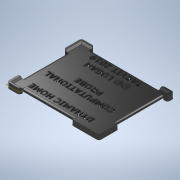
# Autodesk Inventor part: UNO Cover
Saved by Autodesk Inventor 2020.1 (Build 241239000, 239)
## iProperties
Created: 2019-09-15
Part Number: UNO Cover
Material: Generic
Document SubType Name: Modeling
Designer: Logan
Density: 1 g/cm^3
Appearance: Glossy - Black
Author: Logan
Autodesk Inventor part; units mm, degrees
(part 1 of 2)
ref_plane "YZ Plane" through (0, 0, 0) normal (1, 0, 0) x (0, 1, 0)
ref_plane "XZ Plane" through (0, 0, 0) normal (0, 1, 0) x (-1, 0, 0)
ref_plane "XY Plane" through (0, 0, 0) normal (0, 0, 1) x (1, 0, 0)
sketch "Sketch1" plane through (0, 0, 0) normal (0, 1, 0) x (-1, 0, 0)
  line L0 (0, 0) -> (-79.8, 0)
  line L1 (-79.8, 0) -> (-79.8, 63.434)
  line L2 (-79.8, 63.434) -> (0, 63.434)
  line L3 (0, 63.434) -> (0, 0)
  line L4 (-79.8, 0) -> (-73.207, 0)
  line L5 (-73.207, 0) -> (-73.207, 3)
  line L6 (-73.207, 3) -> (-79.8, 3)
  line L7 (-79.8, 3) -> (-79.8, 0)
  line L8 (-79.8, 63.434) -> (-76.8, 63.434)
  line L9 (-76.8, 63.434) -> (-76.8, 47.837)
  line L10 (-76.8, 47.837) -> (-79.8, 47.837)
  line L11 (-79.8, 47.837) -> (-79.8, 63.434)
  line L12 (-79.8, 63.434) -> (-57, 63.434)
  line L13 (-57, 63.434) -> (-57, 60.434)
  line L14 (-57, 60.434) -> (-79.8, 60.434)
  line L15 (-79.8, 60.434) -> (-79.8, 63.434)
  line L16 (-57, 63.434) -> (-31, 63.434)
  line L17 (-31, 63.434) -> (-31, 60.434)
  line L18 (-31, 60.434) -> (-57, 60.434)
  line L19 (-57, 60.434) -> (-57, 63.434)
  line L20 (-31, 60.434) -> (-29.5, 60.434)
  line L21 (-29.5, 60.434) -> (-29.5, 63.434)
  line L22 (-29.5, 63.434) -> (-31, 63.434)
  line L23 (-31, 63.434) -> (-31, 60.434)
  line L24 (0, 63.434) -> (-8.5, 63.434)
  line L25 (-8.5, 63.434) -> (-8.5, 60.434)
  line L26 (-8.5, 60.434) -> (0, 60.434)
  line L27 (0, 60.434) -> (0, 63.434)
  line L28 (0, 63.434) -> (-3, 63.434)
  line L29 (-3, 63.434) -> (-3, 55.505)
  line L30 (-3, 55.505) -> (0, 55.505)
  line L31 (0, 55.505) -> (0, 63.434)
  line L32 (0, 55.505) -> (-3, 55.505)
  line L33 (-3, 55.505) -> (-3, 46.153)
  line L34 (-3, 46.153) -> (0, 46.153)
  line L35 (0, 46.153) -> (0, 55.505)
  line L36 (-3, 46.153) -> (0, 46.153)
  line L37 (0, 46.153) -> (0, 40.598)
  line L38 (0, 40.598) -> (-3, 40.598)
  line L39 (-3, 40.598) -> (-3, 46.153)
  line L40 (0, 0) -> (-4.25, 0)
  line L41 (-4.25, 0) -> (-4.25, 13.458)
  line L42 (-4.25, 13.458) -> (0, 13.458)
  line L43 (0, 13.458) -> (0, 0)
  line L44 (0, 0) -> (-8.939, 0)
  line L45 (-8.939, 0) -> (-8.939, 3)
  line L46 (-8.939, 3) -> (0, 3)
  line L47 (0, 3) -> (0, 0)
  line L48 (-8.939, 0) -> (0, 0)
  line L49 (0, 0) -> (0, -3)
  line L50 (0, -3) -> (-8.939, -3)
  line L51 (-8.939, -3) -> (-8.939, 0)
  line L52 (0, -3) -> (3, -3)
  line L53 (3, -3) -> (3, 13.458)
  line L54 (3, 13.458) -> (0, 13.458)
  line L55 (0, 13.458) -> (0, -3)
  line L56 (0, 40.598) -> (3, 40.598)
  line L57 (3, 40.598) -> (3, 46.153)
  line L58 (3, 46.153) -> (0, 46.153)
  line L59 (0, 46.153) -> (0, 40.598)
  line L60 (0, 55.505) -> (3, 55.505)
  line L61 (3, 55.505) -> (3, 63.434)
  line L62 (3, 63.434) -> (0, 63.434)
  line L63 (0, 63.434) -> (0, 55.505)
  line L64 (-8.5, 63.434) -> (3, 63.434)
  line L65 (3, 63.434) -> (3, 66.434)
  line L66 (3, 66.434) -> (-8.5, 66.434)
  line L67 (-8.5, 66.434) -> (-8.5, 63.434)
  line L68 (-29.5, 63.434) -> (-31, 63.434)
  line L69 (-31, 63.434) -> (-31, 66.434)
  line L70 (-31, 66.434) -> (-29.5, 66.434)
  line L71 (-29.5, 66.434) -> (-29.5, 63.434)
  line L72 (-57, 63.434) -> (-79.8, 63.434)
  line L73 (-79.8, 63.434) -> (-79.8, 66.434)
  line L74 (-79.8, 66.434) -> (-57, 66.434)
  line L75 (-57, 66.434) -> (-57, 63.434)
  line L76 (-79.8, 66.434) -> (-82.8, 66.434)
  line L77 (-82.8, 66.434) -> (-82.8, 47.837)
  line L78 (-82.8, 47.837) -> (-79.8, 47.837)
  line L79 (-79.8, 47.837) -> (-79.8, 66.434)
  line L80 (-79.8, 3) -> (-83.6566, 3)
  line L81 (-83.6566, 3) -> (-83.6566, 0)
  line L82 (-83.6566, 0) -> (-79.8, 0)
  line L83 (-79.8, 0) -> (-79.8, 3)
  line L84 (-83.6566, 0) -> (-73.207, 0)
  line L85 (-73.207, 0) -> (-73.207, -3)
  line L86 (-73.207, -3) -> (-83.6566, -3)
  line L87 (-83.6566, -3) -> (-83.6566, 0)
  dimension "d0" = 79.8
  dimension "d1" = 63.434
  dimension "d2" = 6.593
  dimension "d3" = 3
  dimension "d4" = 3
  dimension "d5" = 15.597
  dimension "d6" = 22.8
  dimension "d7" = 3
  dimension "d8" = 26
  dimension "d9" = 1.5
  dimension "d10" = 8.5
  dimension "d11" = 3
  dimension "d12" = 7.929
  dimension "d13" = 9.352
  dimension "d14" = 5.555
  dimension "d15" = 13.458
  dimension "d16" = 8.939
  dimension "d17" = 3
  dimension "d18" = 3
  dimension "d19" = 3
  dimension "d20" = 3
  dimension "d21" = 3
  dimension "d22" = 11.5
  dimension "d23" = 3
  dimension "d24" = 3
  constraints: 176 end point, 44 parallel, 22 horizontal, 22 perpendicular, 6 point on line
  measures "d0" distance of L1.end L2.end
  measures "d1" distance of L0.end L1.end
  measures "d2" distance of L6.end L5.end
  measures "d3" distance of L5.end L4.end
  measures "d4" distance of L9.end L10.end
  measures "d5" distance of L8.end L9.end
  measures "d6" distance of L13.end L14.end
  measures "d7" distance of L12.end L13.end
  measures "d8" distance of L17.end L18.end
  measures "d9" distance of L22.end L21.end
  measures "d10" distance of L26.end L25.end
  measures "d11" distance of L30.end L29.end
  measures "d12" distance of L29.end L28.end
  measures "d13" distance of L33.end L32.end
  measures "d14" distance of L36.end L37.end
  measures "d15" distance of L40.end L41.end
  measures "d16" distance of L45.end L46.end
  measures "d17" distance of L44.end L45.end
  measures "d18" distance of L48.end L49.end
  measures "d19" distance of L54.end L53.end
  measures "d20" distance of L58.end L57.end
  measures "d21" distance of L62.end L61.end
  measures "d22" distance of L66.end L65.end
  measures "d23" distance of L65.end L64.end
  measures "d24" distance of L78.end L77.end
extrude "Extrusion1" add sketch "Sketch1" against normal mid plane 5 contours L49 L50 L51 L0 | L3 L54 L53 L52 L49 | L85 L86 L87 L82 L0 | L82 L81 L80 L1 | L3 L62 L61 L60 | L78 L77 L76 L73 L1 | L2 L67 L66 L65 L62 | L73 L74 L75 L2
ref_plane "Work Plane1" through (0, 0, 0) normal (0, 1, 0) x (1, 0, 0)
sketch "Sketch2" plane through (0, 0, 0) normal (0, 1, 0) x (1, 0, 0)
  line L0 (0, -63.434) -> (8.5, -63.434) projected
  line L1 (79.8, 0) -> (73.207, 0) projected
  line L2 (0, -63.434) -> (79.8, -63.434)
  line L3 (79.8, -63.434) -> (79.8, 0)
  line L4 (79.8, 0) -> (0, 0)
  line L5 (0, 0) -> (0, -63.434)
  constraints: 8 end point, 2 parallel, 1 horizontal, 1 perpendicular
extrude "Extrusion2" add sketch "Sketch2" against normal mid plane 2
fillet "Fillet1" radius 2 16 edges at (82.8, 0, 66.434) (-3, 0, 66.434) (-3, 0, -3) (83.6566, 0, -3) (82.8, 0, 47.837) (8.5, 0, 66.434) (-3, 0, 55.505) (8.939, 0, -3) (73.207, 0, -3) (83.6566, 0, 3) (57, 0, 66.434) (-3, 0, 13.458) (79.8, 1, 25.4185) (41.073, 1, 0) (0, 1, 34.4815) (32.75, 1, 63.434)
chamfer "Chamfer1" distance 1.5 angle 45 2 edges at (79.8, 2.5, 55.6355) (68.4, 2.5, 63.434)
chamfer "Chamfer2" distance 1.5 angle 45 6 edges at (79.8, 2.5, 1.5) (76.5035, 2.5, 0) (4.4695, 2.5, 0) (0, 2.5, 6.729) (0, 2.5, 59.4695) (4.25, 2.5, 63.434)
sketch "Sketch3" plane through (0, 1, 0) normal (0, 1, 0) x (1, 0, 0)
  line L0 (67.7847, -38.7304) -> (8.3805, -38.7304) construction
  line L1 (8.3805, -38.7304) -> (8.3805, -23.3742) construction
  line L2 (8.3805, -23.3742) -> (67.7847, -23.3742) construction
  line L3 (67.7847, -23.3742) -> (67.7847, -38.7304) construction
  spline S0 degree 2 poles (62.4497, -56.7331) (62.4497, -56.0041) (63.086, -54.8579) (63.5706, -54.5503) knots 0 0 0 1 2 2 2
  spline S1 degree 2 poles (63.5706, -54.5503) (63.9752, -54.289) (64.9275, -54.1373) (65.4627, -54.1373) knots 0 0 0 1 2 2 2
  line L4 (65.4627, -54.1373) -> (67.0893, -54.1373)
  line L5 (67.0893, -54.1373) -> (67.0893, -59.3373)
  line L6 (67.0893, -59.3373) -> (65.4795, -59.3373)
  spline S2 degree 2 poles (65.4795, -59.3373) (64.9317, -59.3373) (63.9752, -59.1982) (63.5538, -58.9285) knots 0 0 0 1 2 2 2
  spline S3 degree 2 poles (63.5538, -58.9285) (63.0439, -58.5998) (62.4497, -57.4874) (62.4497, -56.7331) knots 0 0 0 1 2 2 2
  spline S4 degree 2 poles (63.7897, -56.7415) (63.7897, -57.2556) (64.1437, -57.9888) (64.5061, -58.1953) knots 0 0 0 1 2 2 2
  spline S5 degree 2 poles (64.5061, -58.1953) (64.7716, -58.3386) (65.3531, -58.3681) (65.7577, -58.3681) knots 0 0 0 1 2 2 2
  line L7 (65.7577, -58.3681) -> (65.7829, -58.3681)
  line L8 (65.7829, -58.3681) -> (65.7829, -55.1107)
  line L9 (65.7829, -55.1107) -> (65.7577, -55.1107)
  spline S6 degree 2 poles (65.7577, -55.1107) (65.3194, -55.1107) (64.7168, -55.1402) (64.4429, -55.313) knots 0 0 0 1 2 2 2
  spline S7 degree 2 poles (64.4429, -55.313) (64.1226, -55.5152) (63.7897, -56.2274) (63.7897, -56.7415) knots 0 0 0 1 2 2 2
  line L10 (57.3508, -59.3373) -> (59.146, -56.3075)
  line L11 (59.146, -56.3075) -> (59.146, -54.1373)
  line L12 (59.146, -54.1373) -> (60.4523, -54.1373)
  line L13 (60.4523, -54.1373) -> (60.4523, -56.2443)
  line L14 (60.4523, -56.2443) -> (62.2769, -59.3373)
  line L15 (62.2769, -59.3373) -> (60.7894, -59.3373)
  line L16 (60.7894, -59.3373) -> (59.7739, -57.4832)
  line L17 (59.7739, -57.4832) -> (58.792, -59.3373)
  line L18 (58.792, -59.3373) -> (57.3508, -59.3373)
  line L19 (52.4248, -54.1373) -> (53.6805, -54.1373)
  line L20 (53.6805, -54.1373) -> (55.6863, -57.7613)
  line L21 (55.6863, -57.7613) -> (55.6863, -54.1373)
  line L22 (55.6863, -54.1373) -> (56.8789, -54.1373)
  line L23 (56.8789, -54.1373) -> (56.8789, -59.3373)
  line L24 (56.8789, -59.3373) -> (55.2776, -59.3373)
  line L25 (55.2776, -59.3373) -> (53.6173, -56.358)
  line L26 (53.6173, -56.358) -> (53.6173, -59.3373)
  line L27 (53.6173, -59.3373) -> (52.4248, -59.3373)
  line L28 (52.4248, -59.3373) -> (52.4248, -54.1373)
  line L29 (51.9275, -54.1373) -> (50.1703, -59.3373)
  line L30 (50.1703, -59.3373) -> (48.746, -59.3373)
  line L31 (48.746, -59.3373) -> (46.9888, -54.1373)
  line L32 (46.9888, -54.1373) -> (48.333, -54.1373)
  line L33 (48.333, -54.1373) -> (48.6575, -55.1992)
  line L34 (48.6575, -55.1992) -> (50.2925, -55.1992)
  line L35 (50.2925, -55.1992) -> (50.6212, -54.1373)
  line L36 (50.6212, -54.1373) -> (51.9275, -54.1373)
  line L37 (48.944, -56.1431) -> (49.475, -57.8624)
  line L38 (49.475, -57.8624) -> (50.0102, -56.1431)
  line L39 (50.0102, -56.1431) -> (48.944, -56.1431)
  line L40 (41.1609, -54.1373) -> (42.4588, -54.1373)
  line L41 (42.4588, -54.1373) -> (42.4588, -57.5843)
  line L42 (42.4588, -57.5843) -> (43.4027, -55.3593)
  line L43 (43.4027, -55.3593) -> (44.2961, -55.3593)
  line L44 (44.2961, -55.3593) -> (45.24, -57.5843)
  line L45 (45.24, -57.5843) -> (45.24, -54.1373)
  line L46 (45.24, -54.1373) -> (46.4705, -54.1373)
  line L47 (46.4705, -54.1373) -> (46.4705, -59.3373)
  line L48 (46.4705, -59.3373) -> (44.9661, -59.3373)
  line L49 (44.9661, -59.3373) -> (43.8115, -56.771)
  line L50 (43.8115, -56.771) -> (42.6653, -59.3373)
  line L51 (42.6653, -59.3373) -> (41.1609, -59.3373)
  line L52 (41.1609, -59.3373) -> (41.1609, -54.1373)
  line L53 (37.4948, -54.1373) -> (40.2928, -54.1373)
  line L54 (40.2928, -54.1373) -> (40.2928, -55.0433)
  line L55 (40.2928, -55.0433) -> (39.547, -55.0433)
  line L56 (39.547, -55.0433) -> (39.547, -58.4313)
  line L57 (39.547, -58.4313) -> (40.2928, -58.4313)
  line L58 (40.2928, -58.4313) -> (40.2928, -59.3373)
  line L59 (40.2928, -59.3373) -> (37.4948, -59.3373)
  line L60 (37.4948, -59.3373) -> (37.4948, -58.4313)
  line L61 (37.4948, -58.4313) -> (38.2406, -58.4313)
  line L62 (38.2406, -58.4313) -> (38.2406, -55.0433)
  line L63 (38.2406, -55.0433) -> (37.4948, -55.0433)
  line L64 (37.4948, -55.0433) -> (37.4948, -54.1373)
  spline S8 degree 2 poles (34.3849, -54.0362) (35.5564, -54.0362) (36.9301, -55.452) (36.9301, -56.7331) knots 0 0 0 1 2 2 2
  spline S9 degree 2 poles (36.9301, -56.7331) (36.9301, -57.9678) (35.5521, -59.4384) (34.3807, -59.4384) knots 0 0 0 1 2 2 2
  spline S10 degree 2 poles (34.3807, -59.4384) (34.073, -59.4384) (33.5758, -59.3668) (33.3483, -59.3078) knots 0 0 0 1 2 2 2
  spline S11 degree 2 poles (33.3483, -59.3078) (33.1713, -59.253) (32.7541, -59.0718) (32.6235, -59.0044) knots 0 0 0 1 2 2 2
  line L65 (32.6235, -59.0044) -> (32.6235, -57.7655)
  line L66 (32.6235, -57.7655) -> (32.7541, -57.7655)
  spline S12 degree 2 poles (32.7541, -57.7655) (32.851, -57.8498) (33.1376, -58.0857) (33.3188, -58.1953) knots 0 0 0 1 2 2 2
  spline S13 degree 2 poles (33.3188, -58.1953) (33.5, -58.3091) (33.934, -58.465) (34.1742, -58.465) knots 0 0 0 1 2 2 2
  spline S14 degree 2 poles (34.1742, -58.465) (34.4565, -58.465) (34.9243, -58.288) (35.1392, -58.0647) knots 0 0 0 1 2 2 2
  spline S15 degree 2 poles (35.1392, -58.0647) (35.333, -57.8666) (35.5816, -57.1882) (35.5816, -56.7289) knots 0 0 0 1 2 2 2
  spline S16 degree 2 poles (35.5816, -56.7289) (35.5816, -56.2443) (35.3246, -55.5827) (35.1139, -55.3804) knots 0 0 0 1 2 2 2
  spline S17 degree 2 poles (35.1139, -55.3804) (34.9116, -55.1823) (34.4144, -55.0096) (34.1658, -55.0096) knots 0 0 0 1 2 2 2
  spline S18 degree 2 poles (34.1658, -55.0096) (33.9087, -55.0096) (33.441, -55.1823) (33.2808, -55.2877) knots 0 0 0 1 2 2 2
  spline S19 degree 2 poles (33.2808, -55.2877) (33.1038, -55.393) (32.8384, -55.6164) (32.7414, -55.7049) knots 0 0 0 1 2 2 2
  line L67 (32.7414, -55.7049) -> (32.6235, -55.7049)
  line L68 (32.6235, -55.7049) -> (32.6235, -54.4828)
  spline S20 degree 2 poles (32.6235, -54.4828) (32.7667, -54.4154) (33.1418, -54.2469) (33.344, -54.1879) knots 0 0 0 1 2 2 2
  spline S21 degree 2 poles (33.344, -54.1879) (33.5884, -54.112) (34.0141, -54.0362) (34.3849, -54.0362) knots 0 0 0 1 2 2 2
  line L69 (25.3713, -54.1373) -> (26.6776, -54.1373)
  line L70 (26.6776, -54.1373) -> (26.6776, -56.4423)
  line L71 (26.6776, -56.4423) -> (28.4517, -56.4423)
  line L72 (28.4517, -56.4423) -> (28.4517, -54.1373)
  line L73 (28.4517, -54.1373) -> (29.758, -54.1373)
  line L74 (29.758, -54.1373) -> (29.758, -59.3373)
  line L75 (29.758, -59.3373) -> (28.4517, -59.3373)
  line L76 (28.4517, -59.3373) -> (28.4517, -57.4326)
  line L77 (28.4517, -57.4326) -> (26.6776, -57.4326)
  line L78 (26.6776, -57.4326) -> (26.6776, -59.3373)
  line L79 (26.6776, -59.3373) -> (25.3713, -59.3373)
  line L80 (25.3713, -59.3373) -> (25.3713, -54.1373)
  spline S22 degree 2 poles (19.5602, -56.7373) (19.5602, -55.4731) (20.9087, -54.0277) (22.0802, -54.0277) knots 0 0 0 1 2 2 2
  spline S23 degree 2 poles (22.0802, -54.0277) (23.2559, -54.0277) (24.5959, -55.49) (24.5959, -56.7373) knots 0 0 0 1 2 2 2
  spline S24 degree 2 poles (24.5959, -56.7373) (24.5959, -57.9888) (23.2559, -59.4469) (22.0802, -59.4469) knots 0 0 0 1 2 2 2
  spline S25 degree 2 poles (22.0802, -59.4469) (20.9087, -59.4469) (19.5602, -57.9973) (19.5602, -56.7373) knots 0 0 0 1 2 2 2
  spline S26 degree 2 poles (20.9087, -56.7373) (20.9087, -57.205) (21.0983, -57.8582) (21.2627, -58.0647) knots 0 0 0 1 2 2 2
  spline S27 degree 2 poles (21.2627, -58.0647) (21.427, -58.2796) (21.8484, -58.465) (22.076, -58.465) knots 0 0 0 1 2 2 2
  spline S28 degree 2 poles (22.076, -58.465) (22.3162, -58.465) (22.7081, -58.2922) (22.8893, -58.0731) knots 0 0 0 1 2 2 2
  spline S29 degree 2 poles (22.8893, -58.0731) (23.0494, -57.8708) (23.2474, -57.2008) (23.2474, -56.7373) knots 0 0 0 1 2 2 2
  spline S30 degree 2 poles (23.2474, -56.7373) (23.2474, -56.2569) (23.0578, -55.6248) (22.8935, -55.4099) knots 0 0 0 1 2 2 2
  spline S31 degree 2 poles (22.8935, -55.4099) (22.7291, -55.195) (22.3035, -55.0096) (22.076, -55.0096) knots 0 0 0 1 2 2 2
  spline S32 degree 2 poles (22.076, -55.0096) (21.8442, -55.0096) (21.4144, -55.2076) (21.2585, -55.4183) knots 0 0 0 1 2 2 2
  spline S33 degree 2 poles (21.2585, -55.4183) (21.0899, -55.6459) (20.9087, -56.2485) (20.9087, -56.7373) knots 0 0 0 1 2 2 2
  line L81 (13.4753, -54.1373) -> (14.7732, -54.1373)
  line L82 (14.7732, -54.1373) -> (14.7732, -57.5843)
  line L83 (14.7732, -57.5843) -> (15.7171, -55.3593)
  line L84 (15.7171, -55.3593) -> (16.6105, -55.3593)
  line L85 (16.6105, -55.3593) -> (17.5544, -57.5843)
  line L86 (17.5544, -57.5843) -> (17.5544, -54.1373)
  line L87 (17.5544, -54.1373) -> (18.7849, -54.1373)
  line L88 (18.7849, -54.1373) -> (18.7849, -59.3373)
  line L89 (18.7849, -59.3373) -> (17.2805, -59.3373)
  line L90 (17.2805, -59.3373) -> (16.1259, -56.771)
  line L91 (16.1259, -56.771) -> (14.9797, -59.3373)
  line L92 (14.9797, -59.3373) -> (13.4753, -59.3373)
  line L93 (13.4753, -59.3373) -> (13.4753, -54.1373)
  line L94 (12.3966, -54.1373) -> (12.3966, -59.3373)
  line L95 (12.3966, -59.3373) -> (8.8821, -59.3373)
  line L96 (8.8821, -59.3373) -> (8.8821, -58.347)
  line L97 (8.8821, -58.347) -> (11.0987, -58.347)
  line L98 (11.0987, -58.347) -> (11.0987, -57.4326)
  line L99 (11.0987, -57.4326) -> (9.0549, -57.4326)
  line L100 (9.0549, -57.4326) -> (9.0549, -56.4423)
  line L101 (9.0549, -56.4423) -> (11.0987, -56.4423)
  line L102 (11.0987, -56.4423) -> (11.0987, -55.1276)
  line L103 (11.0987, -55.1276) -> (8.8821, -55.1276)
  line L104 (8.8821, -55.1276) -> (8.8821, -54.1373)
  line L105 (8.8821, -54.1373) -> (12.3966, -54.1373)
  spline S34 degree 2 poles (67.1862, -36.9128) (68.3577, -36.9128) (69.7314, -38.3287) (69.7314, -39.6097) knots 0 0 0 1 2 2 2
  spline S35 degree 2 poles (69.7314, -39.6097) (69.7314, -40.8444) (68.3534, -42.3151) (67.182, -42.3151) knots 0 0 0 1 2 2 2
  spline S36 degree 2 poles (67.182, -42.3151) (66.8743, -42.3151) (66.3771, -42.2435) (66.1495, -42.1845) knots 0 0 0 1 2 2 2
  spline S37 degree 2 poles (66.1495, -42.1845) (65.9726, -42.1297) (65.5554, -41.9485) (65.4248, -41.8811) knots 0 0 0 1 2 2 2
  line L106 (65.4248, -41.8811) -> (65.4248, -40.6422)
  line L107 (65.4248, -40.6422) -> (65.5554, -40.6422)
  spline S38 degree 2 poles (65.5554, -40.6422) (65.6523, -40.7264) (65.9389, -40.9624) (66.1201, -41.072) knots 0 0 0 1 2 2 2
  spline S39 degree 2 poles (66.1201, -41.072) (66.3013, -41.1858) (66.7353, -41.3417) (66.9755, -41.3417) knots 0 0 0 1 2 2 2
  spline S40 degree 2 poles (66.9755, -41.3417) (67.2578, -41.3417) (67.7256, -41.1647) (67.9405, -40.9414) knots 0 0 0 1 2 2 2
  spline S41 degree 2 poles (67.9405, -40.9414) (68.1343, -40.7433) (68.3829, -40.0649) (68.3829, -39.6055) knots 0 0 0 1 2 2 2
  spline S42 degree 2 poles (68.3829, -39.6055) (68.3829, -39.1209) (68.1259, -38.4593) (67.9152, -38.2571) knots 0 0 0 1 2 2 2
  spline S43 degree 2 poles (67.9152, -38.2571) (67.7129, -38.059) (67.2157, -37.8862) (66.9671, -37.8862) knots 0 0 0 1 2 2 2
  spline S44 degree 2 poles (66.9671, -37.8862) (66.71, -37.8862) (66.2423, -38.059) (66.0821, -38.1644) knots 0 0 0 1 2 2 2
  spline S45 degree 2 poles (66.0821, -38.1644) (65.9051, -38.2697) (65.6397, -38.4931) (65.5427, -38.5815) knots 0 0 0 1 2 2 2
  line L108 (65.5427, -38.5815) -> (65.4248, -38.5815)
  line L109 (65.4248, -38.5815) -> (65.4248, -37.3595)
  spline S46 degree 2 poles (65.4248, -37.3595) (65.568, -37.2921) (65.9431, -37.1235) (66.1453, -37.0645) knots 0 0 0 1 2 2 2
  spline S47 degree 2 poles (66.1453, -37.0645) (66.3897, -36.9887) (66.8154, -36.9128) (67.1862, -36.9128) knots 0 0 0 1 2 2 2
  spline S48 degree 2 poles (59.9213, -39.614) (59.9213, -38.3498) (61.2698, -36.9044) (62.4413, -36.9044) knots 0 0 0 1 2 2 2
  spline S49 degree 2 poles (62.4413, -36.9044) (63.617, -36.9044) (64.957, -38.3666) (64.957, -39.614) knots 0 0 0 1 2 2 2
  spline S50 degree 2 poles (64.957, -39.614) (64.957, -40.8655) (63.617, -42.3235) (62.4413, -42.3235) knots 0 0 0 1 2 2 2
  spline S51 degree 2 poles (62.4413, -42.3235) (61.2698, -42.3235) (59.9213, -40.8739) (59.9213, -39.614) knots 0 0 0 1 2 2 2
  spline S52 degree 2 poles (61.2698, -39.614) (61.2698, -40.0817) (61.4594, -40.7349) (61.6238, -40.9414) knots 0 0 0 1 2 2 2
  spline S53 degree 2 poles (61.6238, -40.9414) (61.7881, -41.1563) (62.2095, -41.3417) (62.4371, -41.3417) knots 0 0 0 1 2 2 2
  spline S54 degree 2 poles (62.4371, -41.3417) (62.6773, -41.3417) (63.0692, -41.1689) (63.2504, -40.9498) knots 0 0 0 1 2 2 2
  spline S55 degree 2 poles (63.2504, -40.9498) (63.4105, -40.7475) (63.6085, -40.0775) (63.6085, -39.614) knots 0 0 0 1 2 2 2
  spline S56 degree 2 poles (63.6085, -39.614) (63.6085, -39.1336) (63.4189, -38.5015) (63.2546, -38.2866) knots 0 0 0 1 2 2 2
  spline S57 degree 2 poles (63.2546, -38.2866) (63.0902, -38.0717) (62.6646, -37.8862) (62.4371, -37.8862) knots 0 0 0 1 2 2 2
  spline S58 degree 2 poles (62.4371, -37.8862) (62.2053, -37.8862) (61.7755, -38.0843) (61.6196, -38.295) knots 0 0 0 1 2 2 2
  spline S59 degree 2 poles (61.6196, -38.295) (61.451, -38.5226) (61.2698, -39.1251) (61.2698, -39.614) knots 0 0 0 1 2 2 2
  line L110 (53.8364, -37.014) -> (55.1343, -37.014)
  line L111 (55.1343, -37.014) -> (55.1343, -40.461)
  line L112 (55.1343, -40.461) -> (56.0782, -38.236)
  line L113 (56.0782, -38.236) -> (56.9716, -38.236)
  line L114 (56.9716, -38.236) -> (57.9155, -40.461)
  line L115 (57.9155, -40.461) -> (57.9155, -37.014)
  line L116 (57.9155, -37.014) -> (59.146, -37.014)
  line L117 (59.146, -37.014) -> (59.146, -42.214)
  line L118 (59.146, -42.214) -> (57.6416, -42.214)
  line L119 (57.6416, -42.214) -> (56.487, -39.6477)
  line L120 (56.487, -39.6477) -> (55.3408, -42.214)
  line L121 (55.3408, -42.214) -> (53.8364, -42.214)
  line L122 (53.8364, -42.214) -> (53.8364, -37.014)
  spline S60 degree 2 poles (48.7586, -40.5747) (48.7586, -40.2123) (48.9904, -39.555) (49.2053, -39.3358) knots 0 0 0 1 2 2 2
  spline S61 degree 2 poles (49.2053, -39.3358) (49.3359, -39.1968) (49.6562, -38.9692) (49.8458, -38.8892) knots 0 0 0 1 2 2 2
  spline S62 degree 2 poles (49.8458, -38.8892) (50.0397, -38.8091) (50.4906, -38.7164) (50.7687, -38.7164) knots 0 0 0 1 2 2 2
  line L123 (50.7687, -38.7164) -> (51.4513, -38.7164)
  line L124 (51.4513, -38.7164) -> (51.4513, -37.014)
  line L125 (51.4513, -37.014) -> (52.7577, -37.014)
  line L126 (52.7577, -37.014) -> (52.7577, -42.214)
  line L127 (52.7577, -42.214) -> (50.7392, -42.214)
  spline S63 degree 2 poles (50.7392, -42.214) (50.2925, -42.214) (49.6393, -42.0496) (49.3739, -41.8726) knots 0 0 0 1 2 2 2
  spline S64 degree 2 poles (49.3739, -41.8726) (49.0789, -41.6746) (48.7586, -41.0256) (48.7586, -40.5747) knots 0 0 0 1 2 2 2
  spline S65 degree 2 poles (50.0987, -40.541) (50.0987, -40.7644) (50.3094, -41.0804) (50.4526, -41.1394) knots 0 0 0 1 2 2 2
  spline S66 degree 2 poles (50.4526, -41.1394) (50.638, -41.2195) (50.9752, -41.2448) (51.2659, -41.2448) knots 0 0 0 1 2 2 2
  line L128 (51.2659, -41.2448) -> (51.4513, -41.2448)
  line L129 (51.4513, -41.2448) -> (51.4513, -39.6856)
  line L130 (51.4513, -39.6856) -> (51.3586, -39.6856)
  spline S67 degree 2 poles (51.3586, -39.6856) (51.1774, -39.6856) (50.8487, -39.694) (50.7265, -39.7151) knots 0 0 0 1 2 2 2
  spline S68 degree 2 poles (50.7265, -39.7151) (50.6212, -39.732) (50.3894, -39.8331) (50.3262, -39.8963) knots 0 0 0 1 2 2 2
  spline S69 degree 2 poles (50.3262, -39.8963) (50.1914, -40.0227) (50.0987, -40.305) (50.0987, -40.541) knots 0 0 0 1 2 2 2
  spline S70 degree 2 poles (45.9564, -36.9044) (47.0056, -36.9044) (48.135, -37.9157) (48.135, -38.8934) knots 0 0 0 1 2 2 2
  line L131 (48.135, -38.8934) -> (48.135, -42.214)
  line L132 (48.135, -42.214) -> (46.8286, -42.214)
  line L133 (46.8286, -42.214) -> (46.8286, -38.9692)
  spline S71 degree 2 poles (46.8286, -38.9692) (46.8286, -38.4256) (46.4199, -37.8947) (45.9564, -37.8947) knots 0 0 0 1 2 2 2
  spline S72 degree 2 poles (45.9564, -37.8947) (45.5055, -37.8947) (45.0841, -38.4046) (45.0841, -38.9692) knots 0 0 0 1 2 2 2
  line L134 (45.0841, -38.9692) -> (45.0841, -42.214)
  line L135 (45.0841, -42.214) -> (43.7778, -42.214)
  line L136 (43.7778, -42.214) -> (43.7778, -38.8976)
  spline S73 degree 2 poles (43.7778, -38.8976) (43.7778, -37.9368) (44.8776, -36.9044) (45.9564, -36.9044) knots 0 0 0 1 2 2 2
  line L137 (41.7761, -37.014) -> (41.7761, -41.2237)
  line L138 (41.7761, -41.2237) -> (43.3142, -41.2237)
  line L139 (43.3142, -41.2237) -> (43.3142, -42.214)
  line L140 (43.3142, -42.214) -> (38.9317, -42.214)
  line L141 (38.9317, -42.214) -> (38.9317, -41.2237)
  line L142 (38.9317, -41.2237) -> (40.4698, -41.2237)
  line L143 (40.4698, -41.2237) -> (40.4698, -37.014)
  line L144 (40.4698, -37.014) -> (41.7761, -37.014)
  line L145 (38.957, -37.014) -> (37.1998, -42.214)
  line L146 (37.1998, -42.214) -> (35.7755, -42.214)
  line L147 (35.7755, -42.214) -> (34.0183, -37.014)
  line L148 (34.0183, -37.014) -> (35.3625, -37.014)
  line L149 (35.3625, -37.014) -> (35.687, -38.0759)
  line L150 (35.687, -38.0759) -> (37.322, -38.0759)
  line L151 (37.322, -38.0759) -> (37.6507, -37.014)
  line L152 (37.6507, -37.014) -> (38.957, -37.014)
  line L153 (35.9735, -39.0198) -> (36.5045, -40.7391)
  line L154 (36.5045, -40.7391) -> (37.0397, -39.0198)
  line L155 (37.0397, -39.0198) -> (35.9735, -39.0198)
  line L156 (32.5013, -37.014) -> (32.5013, -41.2237)
  line L157 (32.5013, -41.2237) -> (34.0393, -41.2237)
  line L158 (34.0393, -41.2237) -> (34.0393, -42.214)
  line L159 (34.0393, -42.214) -> (29.6568, -42.214)
  line L160 (29.6568, -42.214) -> (29.6568, -41.2237)
  line L161 (29.6568, -41.2237) -> (31.1949, -41.2237)
  line L162 (31.1949, -41.2237) -> (31.1949, -37.014)
  line L163 (31.1949, -37.014) -> (32.5013, -37.014)
  line L164 (26.5343, -37.014) -> (29.3324, -37.014)
  line L165 (29.3324, -37.014) -> (29.3324, -37.92)
  line L166 (29.3324, -37.92) -> (28.5865, -37.92)
  line L167 (28.5865, -37.92) -> (28.5865, -41.308)
  line L168 (28.5865, -41.308) -> (29.3324, -41.308)
  line L169 (29.3324, -41.308) -> (29.3324, -42.214)
  line L170 (29.3324, -42.214) -> (26.5343, -42.214)
  line L171 (26.5343, -42.214) -> (26.5343, -41.308)
  line L172 (26.5343, -41.308) -> (27.2802, -41.308)
  line L173 (27.2802, -41.308) -> (27.2802, -37.92)
  line L174 (27.2802, -37.92) -> (26.5343, -37.92)
  line L175 (26.5343, -37.92) -> (26.5343, -37.014)
  spline S74 degree 2 poles (20.934, -39.614) (20.934, -38.3498) (22.2825, -36.9044) (23.4539, -36.9044) knots 0 0 0 1 2 2 2
  spline S75 degree 2 poles (23.4539, -36.9044) (24.6296, -36.9044) (25.9696, -38.3666) (25.9696, -39.614) knots 0 0 0 1 2 2 2
  spline S76 degree 2 poles (25.9696, -39.614) (25.9696, -40.8655) (24.6296, -42.3235) (23.4539, -42.3235) knots 0 0 0 1 2 2 2
  spline S77 degree 2 poles (23.4539, -42.3235) (22.2825, -42.3235) (20.934, -40.8739) (20.934, -39.614) knots 0 0 0 1 2 2 2
  spline S78 degree 2 poles (22.2825, -39.614) (22.2825, -40.0817) (22.4721, -40.7349) (22.6364, -40.9414) knots 0 0 0 1 2 2 2
  spline S79 degree 2 poles (22.6364, -40.9414) (22.8008, -41.1563) (23.2222, -41.3417) (23.4497, -41.3417) knots 0 0 0 1 2 2 2
  spline S80 degree 2 poles (23.4497, -41.3417) (23.6899, -41.3417) (24.0818, -41.1689) (24.263, -40.9498) knots 0 0 0 1 2 2 2
  spline S81 degree 2 poles (24.263, -40.9498) (24.4231, -40.7475) (24.6212, -40.0775) (24.6212, -39.614) knots 0 0 0 1 2 2 2
  spline S82 degree 2 poles (24.6212, -39.614) (24.6212, -39.1336) (24.4316, -38.5015) (24.2672, -38.2866) knots 0 0 0 1 2 2 2
  spline S83 degree 2 poles (24.2672, -38.2866) (24.1029, -38.0717) (23.6773, -37.8862) (23.4497, -37.8862) knots 0 0 0 1 2 2 2
  spline S84 degree 2 poles (23.4497, -37.8862) (23.2179, -37.8862) (22.7881, -38.0843) (22.6322, -38.295) knots 0 0 0 1 2 2 2
  spline S85 degree 2 poles (22.6322, -38.295) (22.4637, -38.5226) (22.2825, -39.1251) (22.2825, -39.614) knots 0 0 0 1 2 2 2
  line L176 (15.7045, -37.014) -> (16.9602, -37.014)
  line L177 (16.9602, -37.014) -> (18.9661, -40.638)
  line L178 (18.9661, -40.638) -> (18.9661, -37.014)
  line L179 (18.9661, -37.014) -> (20.1586, -37.014)
  line L180 (20.1586, -37.014) -> (20.1586, -42.214)
  line L181 (20.1586, -42.214) -> (18.5573, -42.214)
  line L182 (18.5573, -42.214) -> (16.897, -39.2347)
  line L183 (16.897, -39.2347) -> (16.897, -42.214)
  line L184 (16.897, -42.214) -> (15.7045, -42.214)
  line L185 (15.7045, -42.214) -> (15.7045, -37.014)
  line L186 (15.2072, -37.014) -> (13.45, -42.214)
  line L187 (13.45, -42.214) -> (12.0257, -42.214)
  line L188 (12.0257, -42.214) -> (10.2685, -37.014)
  line L189 (10.2685, -37.014) -> (11.6128, -37.014)
  line L190 (11.6128, -37.014) -> (11.9372, -38.0759)
  line L191 (11.9372, -38.0759) -> (13.5722, -38.0759)
  line L192 (13.5722, -38.0759) -> (13.9009, -37.014)
  line L193 (13.9009, -37.014) -> (15.2072, -37.014)
  line L194 (12.2238, -39.0198) -> (12.7547, -40.7391)
  line L195 (12.7547, -40.7391) -> (13.2899, -39.0198)
  line L196 (13.2899, -39.0198) -> (12.2238, -39.0198)
  line L197 (6.2821, -37.014) -> (9.7502, -37.014)
  line L198 (9.7502, -37.014) -> (9.7502, -42.214)
  line L199 (9.7502, -42.214) -> (8.4439, -42.214)
  line L200 (8.4439, -42.214) -> (8.4439, -38.0042)
  line L201 (8.4439, -38.0042) -> (6.2821, -38.0042)
  line L202 (6.2821, -38.0042) -> (6.2821, -37.014)
  spline S86 degree 2 poles (45.8953, -32.0131) (45.8953, -31.6507) (46.127, -30.9933) (46.3419, -30.7742) knots 0 0 0 1 2 2 2
  spline S87 degree 2 poles (46.3419, -30.7742) (46.4726, -30.6351) (46.7928, -30.4076) (46.9824, -30.3275) knots 0 0 0 1 2 2 2
  spline S88 degree 2 poles (46.9824, -30.3275) (47.1763, -30.2474) (47.6272, -30.1547) (47.9053, -30.1547) knots 0 0 0 1 2 2 2
  line L203 (47.9053, -30.1547) -> (48.588, -30.1547)
  line L204 (48.588, -30.1547) -> (48.588, -28.4523)
  line L205 (48.588, -28.4523) -> (49.8943, -28.4523)
  line L206 (49.8943, -28.4523) -> (49.8943, -33.6523)
  line L207 (49.8943, -33.6523) -> (47.8758, -33.6523)
  spline S89 degree 2 poles (47.8758, -33.6523) (47.4291, -33.6523) (46.776, -33.488) (46.5105, -33.311) knots 0 0 0 1 2 2 2
  spline S90 degree 2 poles (46.5105, -33.311) (46.2155, -33.1129) (45.8953, -32.464) (45.8953, -32.0131) knots 0 0 0 1 2 2 2
  spline S91 degree 2 poles (47.2353, -31.9794) (47.2353, -32.2027) (47.446, -32.5188) (47.5893, -32.5777) knots 0 0 0 1 2 2 2
  spline S92 degree 2 poles (47.5893, -32.5777) (47.7747, -32.6578) (48.1118, -32.6831) (48.4025, -32.6831) knots 0 0 0 1 2 2 2
  line L208 (48.4025, -32.6831) -> (48.588, -32.6831)
  line L209 (48.588, -32.6831) -> (48.588, -31.1239)
  line L210 (48.588, -31.1239) -> (48.4953, -31.1239)
  spline S93 degree 2 poles (48.4953, -31.1239) (48.3141, -31.1239) (47.9854, -31.1324) (47.8632, -31.1534) knots 0 0 0 1 2 2 2
  spline S94 degree 2 poles (47.8632, -31.1534) (47.7578, -31.1703) (47.526, -31.2714) (47.4628, -31.3346) knots 0 0 0 1 2 2 2
  spline S95 degree 2 poles (47.4628, -31.3346) (47.328, -31.4611) (47.2353, -31.7434) (47.2353, -31.9794) knots 0 0 0 1 2 2 2
  line L211 (40.3918, -28.4523) -> (41.9805, -28.4523)
  line L212 (41.9805, -28.4523) -> (43.4259, -30.3612)
  line L213 (43.4259, -30.3612) -> (43.8978, -30.3612)
  line L214 (43.8978, -30.3612) -> (43.8978, -28.4523)
  line L215 (43.8978, -28.4523) -> (45.1957, -28.4523)
  line L216 (45.1957, -28.4523) -> (45.1957, -33.6523)
  line L217 (45.1957, -33.6523) -> (43.1056, -33.6523)
  spline S96 degree 2 poles (43.1056, -33.6523) (42.6716, -33.6523) (42.0311, -33.5427) (41.7572, -33.3742) knots 0 0 0 1 2 2 2
  spline S97 degree 2 poles (41.7572, -33.3742) (41.479, -33.1972) (41.1504, -32.6452) (41.1504, -32.2238) knots 0 0 0 1 2 2 2
  spline S98 degree 2 poles (41.1504, -32.2238) (41.1504, -31.6296) (41.6897, -30.8837) (42.1406, -30.6646) knots 0 0 0 1 2 2 2
  line L218 (42.1406, -30.6646) -> (40.3918, -28.4523)
  spline S99 degree 2 poles (42.4904, -32.0594) (42.4904, -32.2575) (42.6421, -32.5398) (42.8149, -32.6157) knots 0 0 0 1 2 2 2
  spline S100 degree 2 poles (42.8149, -32.6157) (42.9371, -32.6662) (43.2363, -32.6957) (43.4596, -32.6957) knots 0 0 0 1 2 2 2
  line L219 (43.4596, -32.6957) -> (43.8978, -32.6957)
  line L220 (43.8978, -32.6957) -> (43.8978, -31.2967)
  line L221 (43.8978, -31.2967) -> (43.5228, -31.2967)
  spline S101 degree 2 poles (43.5228, -31.2967) (43.2531, -31.2967) (42.8696, -31.3641) (42.739, -31.4695) knots 0 0 0 1 2 2 2
  spline S102 degree 2 poles (42.739, -31.4695) (42.6126, -31.5706) (42.4904, -31.8403) (42.4904, -32.0594) knots 0 0 0 1 2 2 2
  spline S103 degree 2 poles (35.2719, -31.0523) (35.2719, -29.7881) (36.6204, -28.3427) (37.7918, -28.3427) knots 0 0 0 1 2 2 2
  spline S104 degree 2 poles (37.7918, -28.3427) (38.9675, -28.3427) (40.3076, -29.805) (40.3076, -31.0523) knots 0 0 0 1 2 2 2
  spline S105 degree 2 poles (40.3076, -31.0523) (40.3076, -32.3038) (38.9675, -33.7619) (37.7918, -33.7619) knots 0 0 0 1 2 2 2
  spline S106 degree 2 poles (37.7918, -33.7619) (36.6204, -33.7619) (35.2719, -32.3123) (35.2719, -31.0523) knots 0 0 0 1 2 2 2
  spline S107 degree 2 poles (36.6204, -31.0523) (36.6204, -31.52) (36.81, -32.1732) (36.9743, -32.3797) knots 0 0 0 1 2 2 2
  spline S108 degree 2 poles (36.9743, -32.3797) (37.1387, -32.5946) (37.5601, -32.78) (37.7876, -32.78) knots 0 0 0 1 2 2 2
  spline S109 degree 2 poles (37.7876, -32.78) (38.0278, -32.78) (38.4197, -32.6072) (38.6009, -32.3881) knots 0 0 0 1 2 2 2
  spline S110 degree 2 poles (38.6009, -32.3881) (38.7611, -32.1858) (38.9591, -31.5158) (38.9591, -31.0523) knots 0 0 0 1 2 2 2
  spline S111 degree 2 poles (38.9591, -31.0523) (38.9591, -30.5719) (38.7695, -29.9398) (38.6051, -29.7249) knots 0 0 0 1 2 2 2
  spline S112 degree 2 poles (38.6051, -29.7249) (38.4408, -29.51) (38.0152, -29.3246) (37.7876, -29.3246) knots 0 0 0 1 2 2 2
  spline S113 degree 2 poles (37.7876, -29.3246) (37.5559, -29.3246) (37.126, -29.5226) (36.9701, -29.7333) knots 0 0 0 1 2 2 2
  spline S114 degree 2 poles (36.9701, -29.7333) (36.8016, -29.9609) (36.6204, -30.5635) (36.6204, -31.0523) knots 0 0 0 1 2 2 2
  spline S115 degree 2 poles (30.3416, -30.0452) (30.3416, -29.6575) (30.6366, -29.0717) (30.881, -28.8779) knots 0 0 0 1 2 2 2
  spline S116 degree 2 poles (30.881, -28.8779) (31.176, -28.6461) (31.8755, -28.4523) (32.4191, -28.4523) knots 0 0 0 1 2 2 2
  line L222 (32.4191, -28.4523) -> (34.4966, -28.4523)
  line L223 (34.4966, -28.4523) -> (34.4966, -33.6523)
  line L224 (34.4966, -33.6523) -> (32.6635, -33.6523)
  spline S117 degree 2 poles (32.6635, -33.6523) (32.0904, -33.6523) (31.5004, -33.5638) (31.2434, -33.4247) knots 0 0 0 1 2 2 2
  spline S118 degree 2 poles (31.2434, -33.4247) (30.9611, -33.2773) (30.6871, -32.7716) (30.6871, -32.4429) knots 0 0 0 1 2 2 2
  spline S119 degree 2 poles (30.6871, -32.4429) (30.6871, -32.0636) (31.0664, -31.4695) (31.4035, -31.3304) knots 0 0 0 1 2 2 2
  line L225 (31.4035, -31.3304) -> (31.4035, -31.3051)
  spline S120 degree 2 poles (31.4035, -31.3051) (30.9189, -31.204) (30.3416, -30.5761) (30.3416, -30.0452) knots 0 0 0 1 2 2 2
  spline S121 degree 2 poles (31.6901, -30.0662) (31.6901, -30.3106) (31.8839, -30.5846) (32.0777, -30.6562) knots 0 0 0 1 2 2 2
  spline S122 degree 2 poles (32.0777, -30.6562) (32.1957, -30.7025) (32.6129, -30.711) (32.9585, -30.711) knots 0 0 0 1 2 2 2
  line L226 (32.9585, -30.711) -> (33.1987, -30.711)
  line L227 (33.1987, -30.711) -> (33.1987, -29.4004)
  line L228 (33.1987, -29.4004) -> (33.127, -29.4004)
  spline S123 degree 2 poles (33.127, -29.4004) (32.6213, -29.4004) (32.2337, -29.4131) (32.0314, -29.5016) knots 0 0 0 1 2 2 2
  spline S124 degree 2 poles (32.0314, -29.5016) (31.8544, -29.5816) (31.6901, -29.8766) (31.6901, -30.0662) knots 0 0 0 1 2 2 2
  spline S125 degree 2 poles (32.0145, -32.1858) (32.0145, -32.3123) (32.1452, -32.5777) (32.28, -32.6367) knots 0 0 0 1 2 2 2
  spline S126 degree 2 poles (32.28, -32.6367) (32.4064, -32.6957) (32.7604, -32.7042) (33.1102, -32.7042) knots 0 0 0 1 2 2 2
  line L229 (33.1102, -32.7042) -> (33.1987, -32.7042)
  line L230 (33.1987, -32.7042) -> (33.1987, -31.6001)
  line L231 (33.1987, -31.6001) -> (33.0343, -31.6001)
  spline S127 degree 2 poles (33.0343, -31.6001) (32.7014, -31.6001) (32.4317, -31.6128) (32.2884, -31.6802) knots 0 0 0 1 2 2 2
  spline S128 degree 2 poles (32.2884, -31.6802) (32.1325, -31.756) (32.0145, -32.0131) (32.0145, -32.1858) knots 0 0 0 1 2 2 2
  line L232 (29.5915, -28.4523) -> (29.5915, -33.6523)
  line L233 (29.5915, -33.6523) -> (26.0771, -33.6523)
  line L234 (26.0771, -33.6523) -> (26.0771, -32.662)
  line L235 (26.0771, -32.662) -> (28.2936, -32.662)
  line L236 (28.2936, -32.662) -> (28.2936, -31.7476)
  line L237 (28.2936, -31.7476) -> (26.2499, -31.7476)
  line L238 (26.2499, -31.7476) -> (26.2499, -30.7573)
  line L239 (26.2499, -30.7573) -> (28.2936, -30.7573)
  line L240 (28.2936, -30.7573) -> (28.2936, -29.4426)
  line L241 (28.2936, -29.4426) -> (26.0771, -29.4426)
  line L242 (26.0771, -29.4426) -> (26.0771, -28.4523)
  line L243 (26.0771, -28.4523) -> (29.5915, -28.4523)
  spline S129 degree 2 poles (52.0961, -13.6171) (52.0961, -12.3656) (53.8659, -10.5958) (55.1175, -10.5958) knots 0 0 0 1 2 2 2
  spline S130 degree 2 poles (55.1175, -10.5958) (56.369, -10.5958) (58.1389, -12.3656) (58.1389, -13.6171) knots 0 0 0 1 2 2 2
  spline S131 degree 2 poles (58.1389, -13.6171) (58.1389, -14.8687) (56.369, -16.6385) (55.1175, -16.6385) knots 0 0 0 1 2 2 2
  spline S132 degree 2 poles (55.1175, -16.6385) (53.8659, -16.6385) (52.0961, -14.8687) (52.0961, -13.6171) knots 0 0 0 1 2 2 2
  spline S133 degree 2 poles (52.7619, -13.6171) (52.7619, -14.5906) (54.144, -15.9896) (55.1175, -15.9896) knots 0 0 0 1 2 2 2
  spline S134 degree 2 poles (55.1175, -15.9896) (56.0909, -15.9896) (57.473, -14.5906) (57.473, -13.6171) knots 0 0 0 1 2 2 2
  spline S135 degree 2 poles (57.473, -13.6171) (57.473, -12.6437) (56.0909, -11.2447) (55.1175, -11.2447) knots 0 0 0 1 2 2 2
  spline S136 degree 2 poles (55.1175, -11.2447) (54.144, -11.2447) (52.7619, -12.6437) (52.7619, -13.6171) knots 0 0 0 1 2 2 2
  spline S137 degree 2 poles (54.0092, -12.2982) (54.1019, -12.256) (54.3, -12.1675) (54.439, -12.1296) knots 0 0 0 1 2 2 2
  spline S138 degree 2 poles (54.439, -12.1296) (54.5823, -12.0875) (54.8056, -12.0453) (54.9784, -12.0453) knots 0 0 0 1 2 2 2
  spline S139 degree 2 poles (54.9784, -12.0453) (55.3029, -12.0453) (55.8886, -12.2392) (56.1035, -12.4372) knots 0 0 0 1 2 2 2
  spline S140 degree 2 poles (56.1035, -12.4372) (56.3226, -12.6395) (56.5755, -13.2252) (56.5755, -13.634) knots 0 0 0 1 2 2 2
  spline S141 degree 2 poles (56.5755, -13.634) (56.5755, -14.0217) (56.3269, -14.6116) (56.1077, -14.8181) knots 0 0 0 1 2 2 2
  spline S142 degree 2 poles (56.1077, -14.8181) (55.8928, -15.0204) (55.3029, -15.2353) (54.9784, -15.2353) knots 0 0 0 1 2 2 2
  spline S143 degree 2 poles (54.9784, -15.2353) (54.7129, -15.2353) (54.2199, -15.092) (54.0092, -14.9867) knots 0 0 0 1 2 2 2
  line L244 (54.0092, -14.9867) -> (54.0092, -14.2745)
  line L245 (54.0092, -14.2745) -> (54.0808, -14.2745)
  spline S144 degree 2 poles (54.0808, -14.2745) (54.1483, -14.3251) (54.3042, -14.4346) (54.4306, -14.4979) knots 0 0 0 1 2 2 2
  spline S145 degree 2 poles (54.4306, -14.4979) (54.5401, -14.5526) (54.8183, -14.6285) (54.9615, -14.6285) knots 0 0 0 1 2 2 2
  spline S146 degree 2 poles (54.9615, -14.6285) (55.3324, -14.6285) (55.7327, -14.1228) (55.7327, -13.634) knots 0 0 0 1 2 2 2
  spline S147 degree 2 poles (55.7327, -13.634) (55.7327, -13.1578) (55.3239, -12.6522) (54.9615, -12.6522) knots 0 0 0 1 2 2 2
  spline S148 degree 2 poles (54.9615, -12.6522) (54.8014, -12.6522) (54.5149, -12.7322) (54.4137, -12.787) knots 0 0 0 1 2 2 2
  spline S149 degree 2 poles (54.4137, -12.787) (54.2957, -12.8502) (54.1356, -12.9598) (54.0808, -13.0061) knots 0 0 0 1 2 2 2
  line L246 (54.0808, -13.0061) -> (54.0092, -13.0061)
  line L247 (54.0092, -13.0061) -> (54.0092, -12.2982)
  spline S150 degree 2 poles (45.4549, -13.6171) (45.4549, -12.3656) (47.2248, -10.5958) (48.4763, -10.5958) knots 0 0 0 1 2 2 2
  spline S151 degree 2 poles (48.4763, -10.5958) (49.7278, -10.5958) (51.4977, -12.3656) (51.4977, -13.6171) knots 0 0 0 1 2 2 2
  spline S152 degree 2 poles (51.4977, -13.6171) (51.4977, -14.8687) (49.7278, -16.6385) (48.4763, -16.6385) knots 0 0 0 1 2 2 2
  spline S153 degree 2 poles (48.4763, -16.6385) (47.2248, -16.6385) (45.4549, -14.8687) (45.4549, -13.6171) knots 0 0 0 1 2 2 2
  spline S154 degree 2 poles (46.1207, -13.6171) (46.1207, -14.5906) (47.5029, -15.9896) (48.4763, -15.9896) knots 0 0 0 1 2 2 2
  spline S155 degree 2 poles (48.4763, -15.9896) (49.4497, -15.9896) (50.8319, -14.5906) (50.8319, -13.6171) knots 0 0 0 1 2 2 2
  spline S156 degree 2 poles (50.8319, -13.6171) (50.8319, -12.6437) (49.4497, -11.2447) (48.4763, -11.2447) knots 0 0 0 1 2 2 2
  spline S157 degree 2 poles (48.4763, -11.2447) (47.5029, -11.2447) (46.1207, -12.6437) (46.1207, -13.6171) knots 0 0 0 1 2 2 2
  spline S158 degree 2 poles (47.368, -12.2982) (47.4607, -12.256) (47.6588, -12.1675) (47.7978, -12.1296) knots 0 0 0 1 2 2 2
  spline S159 degree 2 poles (47.7978, -12.1296) (47.9411, -12.0875) (48.1645, -12.0453) (48.3372, -12.0453) knots 0 0 0 1 2 2 2
  spline S160 degree 2 poles (48.3372, -12.0453) (48.6617, -12.0453) (49.2474, -12.2392) (49.4624, -12.4372) knots 0 0 0 1 2 2 2
  spline S161 degree 2 poles (49.4624, -12.4372) (49.6815, -12.6395) (49.9343, -13.2252) (49.9343, -13.634) knots 0 0 0 1 2 2 2
  spline S162 degree 2 poles (49.9343, -13.634) (49.9343, -14.0217) (49.6857, -14.6116) (49.4666, -14.8181) knots 0 0 0 1 2 2 2
  spline S163 degree 2 poles (49.4666, -14.8181) (49.2517, -15.0204) (48.6617, -15.2353) (48.3372, -15.2353) knots 0 0 0 1 2 2 2
  spline S164 degree 2 poles (48.3372, -15.2353) (48.0718, -15.2353) (47.5787, -15.092) (47.368, -14.9867) knots 0 0 0 1 2 2 2
  line L248 (47.368, -14.9867) -> (47.368, -14.2745)
  line L249 (47.368, -14.2745) -> (47.4397, -14.2745)
  spline S165 degree 2 poles (47.4397, -14.2745) (47.5071, -14.3251) (47.663, -14.4346) (47.7894, -14.4979) knots 0 0 0 1 2 2 2
  spline S166 degree 2 poles (47.7894, -14.4979) (47.899, -14.5526) (48.1771, -14.6285) (48.3204, -14.6285) knots 0 0 0 1 2 2 2
  spline S167 degree 2 poles (48.3204, -14.6285) (48.6912, -14.6285) (49.0915, -14.1228) (49.0915, -13.634) knots 0 0 0 1 2 2 2
  spline S168 degree 2 poles (49.0915, -13.634) (49.0915, -13.1578) (48.6828, -12.6522) (48.3204, -12.6522) knots 0 0 0 1 2 2 2
  spline S169 degree 2 poles (48.3204, -12.6522) (48.1602, -12.6522) (47.8737, -12.7322) (47.7726, -12.787) knots 0 0 0 1 2 2 2
  spline S170 degree 2 poles (47.7726, -12.787) (47.6546, -12.8502) (47.4944, -12.9598) (47.4397, -13.0061) knots 0 0 0 1 2 2 2
  line L250 (47.4397, -13.0061) -> (47.368, -13.0061)
  line L251 (47.368, -13.0061) -> (47.368, -12.2982)
  line L252 (39.0539, -11.329) -> (42.522, -11.329)
  line L253 (42.522, -11.329) -> (42.522, -16.529)
  line L254 (42.522, -16.529) -> (41.2157, -16.529)
  line L255 (41.2157, -16.529) -> (41.2157, -12.3193)
  line L256 (41.2157, -12.3193) -> (39.0539, -12.3193)
  line L257 (39.0539, -12.3193) -> (39.0539, -11.329)
  spline S171 degree 2 poles (33.698, -13.929) (33.698, -12.6648) (35.0465, -11.2194) (36.2179, -11.2194) knots 0 0 0 1 2 2 2
  spline S172 degree 2 poles (36.2179, -11.2194) (37.3936, -11.2194) (38.7337, -12.6816) (38.7337, -13.929) knots 0 0 0 1 2 2 2
  spline S173 degree 2 poles (38.7337, -13.929) (38.7337, -15.1805) (37.3936, -16.6385) (36.2179, -16.6385) knots 0 0 0 1 2 2 2
  spline S174 degree 2 poles (36.2179, -16.6385) (35.0465, -16.6385) (33.698, -15.1889) (33.698, -13.929) knots 0 0 0 1 2 2 2
  spline S175 degree 2 poles (35.0465, -13.929) (35.0465, -14.3967) (35.2361, -15.0499) (35.4004, -15.2564) knots 0 0 0 1 2 2 2
  spline S176 degree 2 poles (35.4004, -15.2564) (35.5648, -15.4713) (35.9862, -15.6567) (36.2137, -15.6567) knots 0 0 0 1 2 2 2
  spline S177 degree 2 poles (36.2137, -15.6567) (36.4539, -15.6567) (36.8458, -15.4839) (37.027, -15.2648) knots 0 0 0 1 2 2 2
  spline S178 degree 2 poles (37.027, -15.2648) (37.1871, -15.0625) (37.3852, -14.3925) (37.3852, -13.929) knots 0 0 0 1 2 2 2
  spline S179 degree 2 poles (37.3852, -13.929) (37.3852, -13.4486) (37.1956, -12.8165) (37.0312, -12.6016) knots 0 0 0 1 2 2 2
  spline S180 degree 2 poles (37.0312, -12.6016) (36.8669, -12.3867) (36.4413, -12.2013) (36.2137, -12.2013) knots 0 0 0 1 2 2 2
  spline S181 degree 2 poles (36.2137, -12.2013) (35.982, -12.2013) (35.5521, -12.3993) (35.3962, -12.61) knots 0 0 0 1 2 2 2
  spline S182 degree 2 poles (35.3962, -12.61) (35.2277, -12.8376) (35.0465, -13.4402) (35.0465, -13.929) knots 0 0 0 1 2 2 2
  spline S183 degree 2 poles (28.5823, -11.624) (28.9236, -11.4849) (30.015, -11.2194) (30.546, -11.2194) knots 0 0 0 1 2 2 2
  spline S184 degree 2 poles (30.546, -11.2194) (31.7722, -11.2194) (33.226, -12.6353) (33.226, -13.9332) knots 0 0 0 1 2 2 2
  spline S185 degree 2 poles (33.226, -13.9332) (33.226, -15.1552) (31.7722, -16.6301) (30.5081, -16.6301) knots 0 0 0 1 2 2 2
  spline S186 degree 2 poles (30.5081, -16.6301) (29.8549, -16.6301) (29.0374, -16.3815) (28.6034, -16.1708) knots 0 0 0 1 2 2 2
  line L258 (28.6034, -16.1708) -> (28.6034, -14.9487)
  line L259 (28.6034, -14.9487) -> (28.7213, -14.9487)
  spline S187 degree 2 poles (28.7213, -14.9487) (28.8141, -15.0204) (29.168, -15.2943) (29.3366, -15.387) knots 0 0 0 1 2 2 2
  spline S188 degree 2 poles (29.3366, -15.387) (29.5304, -15.5008) (30.0445, -15.6609) (30.3311, -15.6609) knots 0 0 0 1 2 2 2
  spline S189 degree 2 poles (30.3311, -15.6609) (30.664, -15.6609) (31.216, -15.4502) (31.4309, -15.2353) knots 0 0 0 1 2 2 2
  spline S190 degree 2 poles (31.4309, -15.2353) (31.6374, -15.0246) (31.8776, -14.3799) (31.8776, -13.9543) knots 0 0 0 1 2 2 2
  spline S191 degree 2 poles (31.8776, -13.9543) (31.8776, -13.044) (30.9632, -12.176) (30.1752, -12.176) knots 0 0 0 1 2 2 2
  spline S192 degree 2 poles (30.1752, -12.176) (30.1035, -12.176) (29.9181, -12.1844) (29.8465, -12.1886) knots 0 0 0 1 2 2 2
  line L260 (29.8465, -12.1886) -> (29.8465, -13.2126)
  line L261 (29.8465, -13.2126) -> (30.8536, -13.2126)
  line L262 (30.8536, -13.2126) -> (30.8536, -14.186)
  line L263 (30.8536, -14.186) -> (28.5823, -14.186)
  line L264 (28.5823, -14.186) -> (28.5823, -11.624)
  line L265 (28.1567, -11.329) -> (26.3995, -16.529)
  line L266 (26.3995, -16.529) -> (24.9752, -16.529)
  line L267 (24.9752, -16.529) -> (23.2179, -11.329)
  line L268 (23.2179, -11.329) -> (24.5622, -11.329)
  line L269 (24.5622, -11.329) -> (24.8867, -12.3909)
  line L270 (24.8867, -12.3909) -> (26.5217, -12.3909)
  line L271 (26.5217, -12.3909) -> (26.8504, -11.329)
  line L272 (26.8504, -11.329) -> (28.1567, -11.329)
  line L273 (25.1732, -13.3348) -> (25.7042, -15.0541)
  line L274 (25.7042, -15.0541) -> (26.2393, -13.3348)
  line L275 (26.2393, -13.3348) -> (25.1732, -13.3348)
  line L276 (18.2455, -11.329) -> (19.5013, -11.329)
  line L277 (19.5013, -11.329) -> (21.5071, -14.953)
  line L278 (21.5071, -14.953) -> (21.5071, -11.329)
  line L279 (21.5071, -11.329) -> (22.6996, -11.329)
  line L280 (22.6996, -11.329) -> (22.6996, -16.529)
  line L281 (22.6996, -16.529) -> (21.0983, -16.529)
  line L282 (21.0983, -16.529) -> (19.438, -13.5497)
  line L283 (19.438, -13.5497) -> (19.438, -16.529)
  line L284 (19.438, -16.529) -> (18.2455, -16.529)
  line L285 (18.2455, -16.529) -> (18.2455, -11.329)
  line L286 (60.2648, -2.7673) -> (60.2648, -6.977)
  line L287 (60.2648, -6.977) -> (61.8029, -6.977)
  line L288 (61.8029, -6.977) -> (61.8029, -7.9673)
  line L289 (61.8029, -7.9673) -> (57.4204, -7.9673)
  line L290 (57.4204, -7.9673) -> (57.4204, -6.977)
  line L291 (57.4204, -6.977) -> (58.9585, -6.977)
  line L292 (58.9585, -6.977) -> (58.9585, -2.7673)
  line L293 (58.9585, -2.7673) -> (60.2648, -2.7673)
  line L294 (57.4457, -2.7673) -> (55.6884, -7.9673)
  line L295 (55.6884, -7.9673) -> (54.2641, -7.9673)
  line L296 (54.2641, -7.9673) -> (52.5069, -2.7673)
  line L297 (52.5069, -2.7673) -> (53.8512, -2.7673)
  line L298 (53.8512, -2.7673) -> (54.1756, -3.8292)
  line L299 (54.1756, -3.8292) -> (55.8107, -3.8292)
  line L300 (55.8107, -3.8292) -> (56.1393, -2.7673)
  line L301 (56.1393, -2.7673) -> (57.4457, -2.7673)
  line L302 (54.4622, -4.7731) -> (54.9931, -6.4924)
  line L303 (54.9931, -6.4924) -> (55.5283, -4.7731)
  line L304 (55.5283, -4.7731) -> (54.4622, -4.7731)
  line L305 (47.1847, -2.7673) -> (48.7734, -2.7673)
  line L306 (48.7734, -2.7673) -> (50.2188, -4.6762)
  line L307 (50.2188, -4.6762) -> (50.6907, -4.6762)
  line L308 (50.6907, -4.6762) -> (50.6907, -2.7673)
  line L309 (50.6907, -2.7673) -> (51.9886, -2.7673)
  line L310 (51.9886, -2.7673) -> (51.9886, -7.9673)
  line L311 (51.9886, -7.9673) -> (49.8985, -7.9673)
  spline S193 degree 2 poles (49.8985, -7.9673) (49.4645, -7.9673) (48.8239, -7.8578) (48.55, -7.6892) knots 0 0 0 1 2 2 2
  spline S194 degree 2 poles (48.55, -7.6892) (48.2719, -7.5122) (47.9432, -6.9602) (47.9432, -6.5388) knots 0 0 0 1 2 2 2
  spline S195 degree 2 poles (47.9432, -6.5388) (47.9432, -5.9446) (48.4826, -5.1988) (48.9335, -4.9796) knots 0 0 0 1 2 2 2
  line L312 (48.9335, -4.9796) -> (47.1847, -2.7673)
  spline S196 degree 2 poles (49.2833, -6.3744) (49.2833, -6.5725) (49.435, -6.8548) (49.6077, -6.9307) knots 0 0 0 1 2 2 2
  spline S197 degree 2 poles (49.6077, -6.9307) (49.7299, -6.9813) (50.0291, -7.0107) (50.2525, -7.0107) knots 0 0 0 1 2 2 2
  line L313 (50.2525, -7.0107) -> (50.6907, -7.0107)
  line L314 (50.6907, -7.0107) -> (50.6907, -5.6117)
  line L315 (50.6907, -5.6117) -> (50.3157, -5.6117)
  spline S198 degree 2 poles (50.3157, -5.6117) (50.046, -5.6117) (49.6625, -5.6791) (49.5319, -5.7845) knots 0 0 0 1 2 2 2
  spline S199 degree 2 poles (49.5319, -5.7845) (49.4055, -5.8856) (49.2833, -6.1553) (49.2833, -6.3744) knots 0 0 0 1 2 2 2
  line L316 (42.4567, -7.9673) -> (44.2434, -2.7673)
  line L317 (44.2434, -2.7673) -> (45.6045, -2.7673)
  line L318 (45.6045, -2.7673) -> (47.3912, -7.9673)
  line L319 (47.3912, -7.9673) -> (46.0385, -7.9673)
  line L320 (46.0385, -7.9673) -> (44.905, -4.4402)